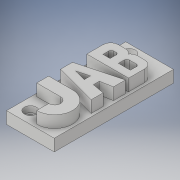
# Autodesk Inventor part: initials
Saved by Autodesk Inventor 2017 (Build 210142000, 142)
## iProperties
Created: 2017-01-30
Part Number: initials
Material: Generic
Document SubType Name: Modeling
Designer: vslabsal
Density: 1 g/cm^3
Appearance: Default
Author: vslabsal
Autodesk Inventor part; units mm, degrees
ref_plane "YZ Plane" through (0, 0, 0) normal (1, 0, 0) x (0, 1, 0)
ref_plane "XZ Plane" through (0, 0, 0) normal (0, 1, 0) x (-1, 0, 0)
ref_plane "XY Plane" through (0, 0, 0) normal (0, 0, 1) x (1, 0, 0)
sketch "Sketch1" plane through (0, 0, 0) normal (0, 1, 0) x (-1, 0, 0)
  line L0 (0, 0) -> (20, 0)
  line L1 (20, 0) -> (20, -50)
  line L2 (20, -50) -> (0, -50)
  line L3 (0, -50) -> (0, 0)
  dimension "d0" = 50
  dimension "d1" = 20
  constraints: 8 end point, 2 parallel, 1 horizontal, 1 perpendicular
  measures "d0" distance of L2.end L0.start
  measures "d1" distance of L0.start L0.end
extrude "Extrusion1" add sketch "Sketch1" along normal blind 10
sketch "Sketch4" plane through (0, 10, 0) normal (0, 1, 0) x (1, 0, 0)
  line L0 (-18.73, 16.39) -> (-18.73, 11.39)
  line L1 (-18.73, 11.39) -> (-8.73, 11.39)
  line L2 (-8.73, 11.39) -> (-8.73, 6.39) construction
  line L3 (-18.73, 16.39) -> (-8.73, 16.39)
  arc A0 (-8.73, 6.39) -> (-8.73, 11.39) centre (-8.73, 8.89) ccw
  line L4 (-8.73, 6.39) -> (-8.73, 1.39)
  arc A1 (-15.8011, 11.39) -> (-8.73, 1.39) centre (-8.73, 8.89) ccw construction
  line L5 (-20, 0) -> (0, 0) construction
  line L6 (0, 0) -> (0, 50) construction
  line L7 (0, 50) -> (-20, 50) construction
  line L8 (-20, 50) -> (-20, 0) construction
  line L9 (-20, 0) -> (0, 0) projected
  line L10 (-10, 0) -> (-10, 50) construction
  arc A2 (-10, 16.2817) -> (-15.8011, 11.39) centre (-8.73, 8.89) ccw construction
  arc A3 (-8.73, 1.39) -> (-10, 16.2817) centre (-8.73, 8.89) ccw
  arc A4 (-10, 6.7366) -> (-8.73, 6.39) centre (-8.73, 8.89) ccw construction
  arc A5 (-8.73, 11.39) -> (-10, 6.7366) centre (-8.73, 8.89) ccw construction
  line L11 (-1.23, 8.89) -> (-1.23, 50) construction
  line L12 (-1.23, 16.7009) -> (-18.73, 21.39)
  line L13 (-18.73, 21.39) -> (-18.73, 26.39)
  line L14 (-18.73, 26.39) -> (-1.23, 31.0791)
  line L15 (-1.23, 32.39) -> (-18.73, 32.39)
  line L16 (-1.23, 16.7009) -> (-1.23, 21.7009)
  line L17 (-6.23, 22.64) -> (-1.23, 21.7009)
  line L18 (-6.23, 22.64) -> (-6.23, 25.14)
  line L19 (-6.23, 25.14) -> (-1.23, 26.0791)
  line L20 (-1.23, 31.0791) -> (-1.23, 26.0791)
  line L21 (-18.73, 23.89) -> (-1.23, 23.89) construction
  line L22 (-14.98, 23.89) -> (-9.98, 22.5503)
  line L23 (-9.98, 22.5503) -> (-9.98, 25.2297)
  line L24 (-9.98, 25.2297) -> (-14.98, 23.89)
  line L25 (-1.23, 32.39) -> (-1.23, 42.39)
  line L26 (-1.23, 42.39) -> (-9.375, 42.39)
  line L27 (-10, 42.39) -> (-10, 42.39)
  line L28 (-10, 42.39) -> (-10.625, 42.39)
  line L29 (-18.73, 42.39) -> (-18.73, 32.39)
  line L30 (-8.73, 35.64) -> (-3.73, 35.64)
  line L31 (-3.73, 35.64) -> (-3.73, 39.14)
  line L32 (-3.73, 39.14) -> (-8.73, 39.14)
  line L33 (-8.73, 39.14) -> (-8.73, 35.64)
  line L34 (-6.23, 32.39) -> (-6.23, 42.39) construction
  line L35 (-6.23, 37.39) -> (-1.23, 37.39) construction
  line L36 (-6.23, 37.39) -> (-10, 37.39) construction
  line L37 (-15.23, 35.64) -> (-12.23, 35.64)
  line L38 (-12.23, 35.64) -> (-12.23, 39.14)
  line L39 (-12.23, 39.14) -> (-15.23, 39.14)
  line L40 (-15.23, 39.14) -> (-15.23, 35.64)
  line L41 (-12.23, 37.39) -> (-10, 37.39) construction
  line L42 (-20, 50) -> (-20, 0) projected
  line L43 (-20, 0) -> (-20, 50)
  line L44 (0, 50) -> (-20, 50) projected
  line L45 (-20, 50) -> (0, 50)
  line L46 (0, 50) -> (0, 0)
  line L47 (-10.625, 42.39) -> (-10, 41.14)
  line L48 (-10, 41.14) -> (-9.375, 42.39)
  line L49 (-10, 42.39) -> (-10.625, 42.39)
  line L50 (-10, 42.39) -> (-9.375, 42.39)
  line L51 (-10.625, 42.39) -> (-18.73, 42.39)
  line L52 (-9.375, 42.39) -> (-10, 42.39)
  point P0 (-6.23, 23.89)
  point P1 (-9.98, 23.89)
  point P2 (-6.23, 39.14)
  point P3 (-8.73, 37.39)
  dimension "d11" = 5
  dimension "d12" = 10
  dimension "d14" = 5
  dimension "d16" = 10
  dimension "d17" = 1.27
  dimension "d18" = 8.89
  dimension "d19" = 75
  dimension "d20" = 75
  dimension "d21" = 5
  dimension "d22" = 2.5
  dimension "d23" = 15
  dimension "d24" = 5
  dimension "d25" = 5
  dimension "d26" = 8.5
  dimension "d27" = 10
  dimension "d28" = 10
  dimension "d29" = 5
  dimension "d34" = 3.5
  dimension "d35" = 1.25
  dimension "d36" = 1.25
  dimension "d39" = 2.5
  dimension "d40" = 3.5
  dimension "d41" = 3.5
  constraints: 92 end point, 21 point on line, 15 point on circle, 13 midpoint, 12 perpendicular, 11 collinear, 8 horizontal, 6 centre point, 6 parallel, 6 vertical, 4 equal length, 3 tangent
  measures "d11" distance between parallel lines of L3 L1
  measures "d12" distance from line of A1.centre L0
  measures "d14" diameter of A0
  measures "d16" distance between parallel lines of L6 L10
  measures "d17" distance from line of A0.centre L10
  measures "d18" distance from line of L5 A0.centre
  measures "d19" angle of L11 L12
  measures "d20" angle of L20 L14
  measures "d21" distance of L12.end L13.end
  measures "d22" distance of L17.start L18.end
  measures "d23" distance from line of L21 A0.centre
  measures "d24" distance between parallel lines of L20 L18
  measures "d25" distance from line of L23 L22.start
  measures "d26" distance from line of L15 point (-9.98, 23.89)
  measures "d27" distance of L29.start L15.end
  measures "d28" distance of L25.start L25.end
  measures "d29" distance between parallel lines of L11 L34
  measures "d34" distance between parallel lines of L33 L38
  measures "d35" distance of L27.start L47.end
  measures "d36" distance of L26.end L28.end
  measures "d39" distance between parallel lines of L11 L31
  measures "d40" distance between parallel lines of L32 L30
  measures "d41" distance between parallel lines of L29 L40
extrude "Extrusion3" cut sketch "Sketch4" against normal blind 5 contours L42 L44 L46 L9 | L48 L47 L28 L50 | L24 L23 L22 | L33 L32 L31 L30 | L40 L39 L38 L37
fillet "Fillet1" radius 3.175 4 edges at (-18.73, 7.5, -42.39) (-10.625, 7.5, -42.39) (-9.375, 7.5, -42.39) (-1.23, 7.5, -42.39)
sketch "Sketch5" plane through (0, 5, 0) normal (0, 1, 0) x (1, 0, 0)
  line L0 (-20, 50) -> (0, 50) projected
  line L1 (-20, 0) -> (-20, 50) projected
  line L2 (0, 0) -> (-20, 0) projected
  point P0 (-15, 5)
  point P1 (-15, 46.5)
  dimension "d43" = 3.5
  dimension "d44" = 5
  dimension "d45" = 5
  dimension "d46" = 5
  measures "d43" distance from line of L0 point (-15, 46.5)
  measures "d44" horizontal distance of L0.start point (-15, 46.5)
  measures "d45" distance from line of point (-15, 5) L1
  measures "d46" distance from line of L2 point (-15, 5)
hole "Hole1" at (-15, 5, -5) at (-15, 5, -46.5) direction (0, -1, 0) diameter 3.175 end through all counterbore diameter 5.08 counterbore depth 2.54
fillet "Fillet2" radius 0.9525 4 edges at (-8.73, 7.5, -39.14) (-3.73, 7.5, -39.14) (-12.23, 7.5, -39.14) (-15.23, 7.5, -39.14)
equation "\"d20\" = d19"
equation "\"d22\" = 0.5 * d21"
body "Solid1"
